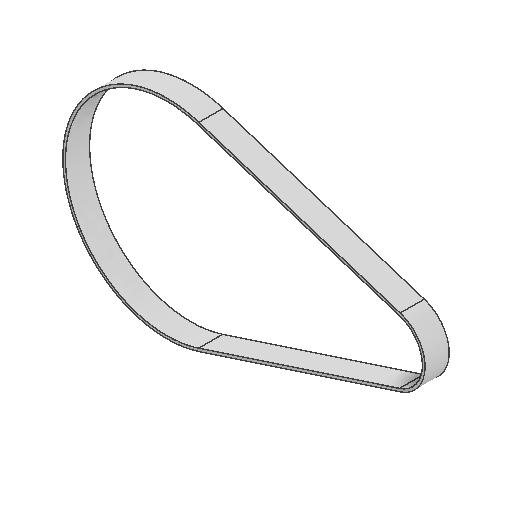
# Autodesk Inventor part: Diff Motor Belts
Saved by Autodesk Inventor 2025.2 (Build 292293000, 293)
## iProperties
Created: 2025-02-20
Part Number: Diff Motor Belts
Material: Generic
Document SubType Name: Modeling
Designer: Jakeg
Density: 1 g/cm^3
Appearance: Default
Author: Jakeg
Autodesk Inventor part; units mm, degrees
ref_plane "YZ Plane" through (0, 0, 0) normal (1, 0, 0) x (0, 1, 0)
ref_plane "XZ Plane" through (0, 0, 0) normal (0, 1, 0) x (-1, 0, 0)
ref_plane "XY Plane" through (0, 0, 0) normal (0, 0, 1) x (1, 0, 0)
sketch "Sketch1" plane through (0, 0, 0) normal (0, 0, 1) x (1, 0, 0)
  circle A0 centre (0, 0) radius 38.3032
  circle A1 centre (83.8197, 0.2342) radius 12.4968
  circle A2 centre (0, 0) radius 39.3192
  circle A3 centre (83.8197, 0.2342) radius 13.5128
  line L0 (12.21, -37.3753) -> (88.0159, -12.6105)
  line L1 (11.8945, -36.4095) -> (87.7004, -11.6448)
  line L2 (87.6339, 12.1347) -> (11.6909, 36.4755)
  line L3 (87.944, 13.1022) -> (12.001, 37.443)
  point P0 (17.6469, -33.9959)
  point P1 (17.4567, 34.094)
  dimension "d0" = 76.6064
  dimension "d1" = 24.9936
  dimension "d2" = 83.82
  dimension "d3" = 78.6384
  dimension "d4" = 27.0256
  dimension "d5" = 1.016
  dimension "d6" = 1.016
  constraints: 8 end point, 8 point on circle, 4 centre point, 4 tangent, 3 coincident, 2 parallel
  measures "d0" diameter of A0
  measures "d1" diameter of A1
  measures "d2" distance of A1.centre point (0, 0)
  measures "d3" diameter of A2
  measures "d4" diameter of A3
  measures "d5" distance between parallel lines of L3 L2
  measures "d6" distance between parallel lines of L1 L0
extrude "Extrusion1" add sketch "Sketch1" along normal blind 9.0932 contours A0 L1 A2 L2 | A2 L3 A3 L2 | L1 A3 L0 A2 | A3 L1 A1 L2 picked at (0.5493, 38.7633) picked at (85.0283, -12.7145)
body "Solid1"
